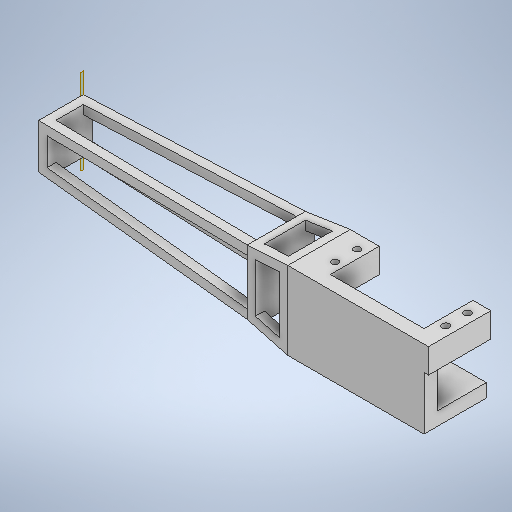
# Autodesk Inventor part: tibiaModel
Saved by Autodesk Inventor 2025.1 (Build 291241020, 241B)
## iProperties
Created: 2021-12-15
Part Number: tibiaModel
Material: 钢
Document SubType Name: Modeling
Designer: omiye
Density: 7.85 g/cm^3
Appearance: Default
Mass: 171.923 g
Surface Area: 96.234 cm^2
Volume: 21.901 cm^3
Sending System: Autodesk Translation Framework v10.10.0.1391
Preprocessor: ST-DEVELOPER v18.1
Title: C:/Users/23714/Desktop/Servo Motor MG996R_ 一字摇臂.step
Autodesk Inventor part; units mm, degrees
ref_plane "YZ Plane" through (0, 0, 0) normal (1, 0, 0) x (0, 1, 0)
ref_plane "XZ Plane" through (0, 0, 0) normal (0, 1, 0) x (-1, 0, 0)
ref_plane "XY Plane" through (0, 0, 0) normal (0, 0, 1) x (1, 0, 0)
ref_plane "Work Plane1" through (-19.25, -0.5, 9.85) normal (0, 0, 1) x (1, 0, 0)
sketch "Sketch1" plane through (-19.25, -0.5, 9.85) normal (0, 0, 1) x (1, 0, 0)
  line L0 (-0.695, -27.8) -> (39.2, -27.8)
  line L1 (39.2, -27.8) -> (39.2, 8.9608)
  line L2 (39.2, 8.9608) -> (-0.695, 8.9608)
  line L3 (-0.695, 8.9608) -> (-0.695, -27.8)
  point P0 (19.25, 0.5)
  constraints: 8 end point, 2 parallel, 1 horizontal, 1 perpendicular
extrude "Extrusion1" add sketch "Sketch1" along normal blind 3
ref_plane "Work Plane2" through (-19.25, -0.5, 12.85) normal (0, 0, 1) x (1, 0, 0)
sketch "Sketch2" plane through (-19.25, -0.5, 12.85) normal (0, 0, 1) x (1, 0, 0)
  line L0 (39.2, -27.8) -> (39.2, 8.9608) projected
  line L1 (39.2, -27.8) -> (-0.695, -27.8)
  line L2 (-0.695, -27.8) -> (-0.695, 8.9608)
  line L3 (-0.695, 8.9608) -> (39.2, 8.9608)
  line L4 (39.2, 8.9608) -> (39.2, -27.8)
  point P0 (19.25, 0.5)
  point P1 (39.2, 8.9608)
  constraints: 8 end point, 2 parallel, 1 horizontal, 1 perpendicular
extrude "Extrusion2" add sketch "Sketch2" along normal blind 5
ref_plane "Work Plane4" through (19.95, -28.3, 9.85) normal (1, 0, 0) x (0, 0, -1)
sketch "Sketch3" plane through (19.95, -28.3, 9.85) normal (1, 0, 0) x (0, 0, -1)
  line L0 (0, 0) -> (0, 36.7608) projected
  line L1 (0, 0) -> (-8, 0) projected
  line L2 (0, 36.7608) -> (-2, 36.7608)
  line L3 (-2, 36.7608) -> (-2, 0)
  line L4 (-2, 0) -> (0, 0)
  line L5 (0, 0) -> (0, 36.7608)
  point P0 (9.85, 28.3)
  dimension "d4" = 2
  constraints: 8 end point, 2 parallel, 1 horizontal, 1 perpendicular, 1 point on line
  measures "d4" distance of L4.end L3.end
extrude "Extrusion3" cut sketch "Sketch3" against normal blind 50
ref_plane "Work Plane3" through (19.95, -28.3, 17.85) normal (1, 0, 0) x (0, 0, -1)
sketch "Sketch4" plane through (19.95, -28.3, 17.85) normal (1, 0, 0) x (0, 0, -1)
  line L0 (6, 0) -> (0, 0) projected
  line L1 (6, 36.7608) -> (0, 36.7608) projected
  line L2 (0, 0) -> (1, 0)
  line L3 (1, 0) -> (1, 36.7608)
  line L4 (1, 36.7608) -> (0, 36.7608)
  line L5 (0, 36.7608) -> (0, 0)
  point P0 (17.85, 28.3)
  point P1 (1, 0)
  dimension "d7" = 1
  constraints: 8 end point, 2 parallel, 1 horizontal, 1 perpendicular, 1 point on line
  measures "d7" distance of L4.end L3.end
extrude "Extrusion4" cut sketch "Sketch4" against normal blind 50
ref_plane "Work Plane5" through (19.95, -28.3, 11.85) normal (1, 0, 0) x (0, 0, -1)
sketch "Sketch5" plane through (19.95, -28.3, 11.85) normal (1, 0, 0) x (0, 0, -1)
  line L0 (-5, 36.7608) -> (-5, 0) projected
  line L1 (0, 0) -> (0, 36.7608) projected
  line L2 (-5, 36.7608) -> (0, 36.7608)
  line L3 (0, 36.7608) -> (0, 0)
  line L4 (0, 0) -> (-5, 0)
  line L5 (-5, 0) -> (-5, 36.7608)
  point P0 (11.85, 28.3)
  constraints: 8 end point, 2 parallel, 1 horizontal, 1 perpendicular
extrude "Extrusion5" add sketch "Sketch5" along normal blind 7
ref_plane "Work Plane6" through (-19.945, -28.3, 11.85) normal (0, 0, -1) x (-1, 0, 0)
sketch "Sketch6" plane through (-19.945, -28.3, 11.85) normal (0, 0, -1) x (-1, 0, 0)
  line L0 (-46.895, 0) -> (-46.895, 36.7608) projected
  line L1 (-46.895, 27.8459) -> (-40.895, 27.8459)
  line L2 (-40.895, 27.8459) -> (-40.895, 11.8459)
  line L3 (-40.895, 11.8459) -> (-46.895, 11.8459)
  line L4 (-46.895, 11.8459) -> (-46.895, 27.8459)
  point P0 (-19.945, 28.3)
  dimension "d12" = 6
  dimension "d13" = 16
  constraints: 8 end point, 2 parallel, 1 horizontal, 1 perpendicular, 1 point on line
  measures "d12" distance of L2.end L3.end
  measures "d13" distance of L1.end L2.end
extrude "Extrusion6" add sketch "Sketch6" along normal blind 22.875
sketch "Sketch7" plane through (20.95, -0.4541, 11.85) normal (0, 1, 0) x (1, 0, 0)
  arc A0 (5.4164, 8.2173) -> (5.4164, 5.6327) centre (3.7611, 6.925) ccw projected
  circle A1 centre (3.7611, 6.925) radius 2.5
  arc A2 (5.4164, 18.0673) -> (5.4164, 15.4827) centre (3.7611, 16.775) ccw projected
  circle A3 centre (3.7611, 16.775) radius 2.5
  point P0 (-20.95, 11.85)
  dimension "d16" = 5
  dimension "d17" = 5
  constraints: 2 centre point, 2 coincident
  measures "d16" diameter of A1
  measures "d17" diameter of A3
extrude "Extrusion7" cut sketch "Sketch7" against normal blind 22.875
ref_plane "Work Plane7" through (26.95, -28.3, 11.85) normal (1, 0, 0) x (0, 0, -1)
sketch "Sketch8" plane through (26.95, -28.3, 11.85) normal (1, 0, 0) x (0, 0, -1)
  line L0 (0, 11.8459) -> (22.875, 11.8459) projected
  line L1 (22.875, 27.8459) -> (22.875, 11.8459) projected
  line L2 (0, 11.8459) -> (22.875, 11.8459)
  line L3 (22.875, 11.8459) -> (22.875, 16.8459)
  line L4 (22.875, 16.8459) -> (0, 16.8459)
  line L5 (0, 16.8459) -> (0, 11.8459)
  point P0 (11.85, 28.3)
  dimension "d20" = 5
  constraints: 8 end point, 2 parallel, 1 horizontal, 1 perpendicular, 1 point on line
  measures "d20" distance of L3.end L2.end
extrude "Extrusion8" cut sketch "Sketch8" against normal blind 6.7
ref_plane "Work Plane8" through (-19.945, -28.3, 11.85) normal (-1, 0, 0) x (0, 0, 1)
sketch "Sketch9" plane through (-19.945, -28.3, 11.85) normal (-1, 0, 0) x (0, 0, 1)
  line L0 (0, 36.7608) -> (0, 0) projected
  line L1 (5, 0) -> (0, 0) projected
  line L2 (0, 36.7608) -> (5, 36.7608)
  line L3 (5, 36.7608) -> (5, 0)
  line L4 (5, 0) -> (0, 0)
  line L5 (0, 0) -> (0, 36.7608)
  point P0 (-11.85, 28.3)
  constraints: 8 end point, 2 parallel, 1 horizontal, 1 perpendicular
extrude "Extrusion9" add sketch "Sketch9" along normal blind 7
ref_plane "Work Plane10" through (26.95, -0.4541, 11.85) normal (0, 0, -1) x (-1, 0, 0)
sketch "Sketch11" plane through (26.95, -0.4541, 11.85) normal (0, 0, -1) x (-1, 0, 0)
  line L0 (53.895, -27.8459) -> (53.895, 8.9148) projected
  line L1 (53.895, 0) -> (47.895, 0)
  line L2 (47.895, 0) -> (47.895, -11)
  line L3 (47.895, -11) -> (53.895, -11)
  line L4 (53.895, -11) -> (53.895, 0)
  point P0 (26.95, 0.4541)
  dimension "d25" = 6
  constraints: 8 end point, 2 parallel, 1 horizontal, 1 perpendicular, 1 point on line
  measures "d25" distance of L3.end L2.end
extrude "Extrusion10" add sketch "Sketch11" along normal blind 22.875
sketch "Sketch12" plane through (-26.945, -0.4541, 11.85) normal (0, 1, 0) x (1, 0, 0)
  arc A0 (0.5786, 15.4827) -> (0.5786, 18.0673) centre (2.2339, 16.775) ccw projected
  circle A1 centre (2.2339, 16.775) radius 2.5
  arc A2 (0.5786, 5.6327) -> (0.5786, 8.2173) centre (2.2339, 6.925) ccw projected
  circle A3 centre (2.2339, 6.925) radius 2.5
  point P0 (26.945, 11.85)
  dimension "d28" = 5
  dimension "d29" = 5
  constraints: 2 centre point, 2 coincident
  measures "d28" diameter of A1
  measures "d29" diameter of A3
extrude "Extrusion11" cut sketch "Sketch12" against normal blind 22.875
ref_plane "Work Plane11" through (-26.945, -28.3, 11.85) normal (-1, 0, 0) x (0, 0, 1)
sketch "Sketch13" plane through (-26.945, -28.3, 11.85) normal (-1, 0, 0) x (0, 0, 1)
  line L0 (0, 16.8459) -> (0, 27.8459) projected
  line L1 (5, 36.7608) -> (0, 36.7608) projected
  line L2 (0, 27.8459) -> (5, 27.8459)
  line L3 (5, 27.8459) -> (5, 36.7608)
  line L4 (5, 36.7608) -> (0, 36.7608)
  line L5 (0, 36.7608) -> (0, 27.8459)
  point P0 (-11.85, 28.3)
  constraints: 8 end point, 2 parallel, 1 horizontal, 1 perpendicular
extrude "Extrusion12" cut sketch "Sketch13" against normal blind 67.325
ref_plane "Work Plane9" through (26.95, -28.3, 11.85) normal (0, -1, 0) x (1, 0, 0)
sketch "Sketch14" plane through (26.95, -28.3, 11.85) normal (0, -1, 0) x (1, 0, 0)
  line L0 (0, 5) -> (0, 0) projected
  line L1 (0, 5) -> (-53.895, 5) projected
  line L2 (0, 0) -> (-53.895, 0)
  line L3 (-53.895, 0) -> (-53.895, 5)
  line L4 (-53.895, 5) -> (0, 5)
  line L5 (0, 5) -> (0, 0)
  point P0 (-26.95, -11.85)
  constraints: 8 end point, 2 parallel, 1 horizontal, 1 perpendicular
extrude "Extrusion13" add sketch "Sketch14" along normal blind 5
ref_plane "Work Plane12" through (26.95, -11.4541, 11.85) normal (0, 0, -1) x (-1, 0, 0)
sketch "Sketch15" plane through (26.95, -11.4541, 11.85) normal (0, 0, -1) x (-1, 0, 0)
  line L0 (53.895, -21.8459) -> (0, -21.8459) projected
  line L1 (53.895, 11) -> (53.895, -21.8459) projected
  line L2 (0, -21.8459) -> (53.895, -21.8459)
  line L3 (53.895, -21.8459) -> (53.895, -17.8459)
  line L4 (53.895, -17.8459) -> (0, -17.8459)
  line L5 (0, -17.8459) -> (0, -21.8459)
  point P0 (26.95, 11.4541)
  dimension "d36" = 4
  constraints: 8 end point, 2 parallel, 1 horizontal, 1 perpendicular, 1 point on line
  measures "d36" distance of L3.end L2.end
extrude "Extrusion14" add sketch "Sketch15" along normal blind 22.4625
ref_plane "Work Plane13" through (-26.945, -29.3, 11.85) normal (0, 1, 0) x (1, 0, 0)
sketch "Sketch16" plane through (-26.945, -29.3, 11.85) normal (0, 1, 0) x (1, 0, 0)
  line L0 (53.895, 0) -> (53.895, 22.4625) projected
  line L1 (0, 0) -> (0, 22.4625) projected
  line L2 (53.895, 0) -> (0, 0)
  line L3 (0, 0) -> (0, 1)
  line L4 (0, 1) -> (53.895, 1)
  line L5 (53.895, 1) -> (53.895, 0)
  point P0 (26.945, 11.85)
  point P1 (53.895, 1)
  dimension "d39" = 1
  constraints: 8 end point, 2 parallel, 1 horizontal, 1 perpendicular, 1 point on line
  measures "d39" distance of L2.end L3.end
extrude "Extrusion15" add sketch "Sketch16" along normal blind 30
ref_plane "Work Plane14" through (26.95, -28.3, 11.85) normal (1, 0, 0) x (0, 0, -1)
sketch "Sketch17" plane through (26.95, -28.3, 11.85) normal (1, 0, 0) x (0, 0, -1)
  line L0 (0, 29) -> (1, 29) projected
  line L1 (5.8126, 27.8459) -> (1, 27.8459) projected
  line L2 (0, 29) -> (1, 29)
  line L3 (1, 29) -> (1, 27.8459)
  line L4 (1, 27.8459) -> (0, 27.8459)
  line L5 (0, 27.8459) -> (0, 29)
  point P0 (11.85, 28.3)
  constraints: 8 end point, 2 parallel, 1 horizontal, 1 perpendicular
extrude "Extrusion16" cut sketch "Sketch17" against normal blind 100
sketch "Sketch19" plane through (26.95, -33.3, 11.85) normal (0, -1, 0) x (1, 0, 0)
  circle A0 centre (-16.85, -11.85) radius 5
  circle A1 centre (-16.85, -11.85) radius 1.5
  point P0 (-26.95, -11.85)
  dimension "d47" = 10
  dimension "d50" = 3
  constraints: 2 centre point, 1 coincident
  measures "d47" diameter of A0
  measures "d50" diameter of A1
extrude "Extrusion20" cut sketch "Sketch19" against normal blind 10 contours A1
sketch "Sketch20" plane through (26.95, -33.3, 11.85) normal (0, -1, 0) x (1, 0, 0)
  line L0 (-53.895, -22.4625) -> (0, -22.4625) projected
  line L1 (-53.895, 5) -> (-53.895, -22.4625) projected
  line L2 (0, -22.4625) -> (-53.895, -22.4625)
  line L3 (-53.895, -22.4625) -> (-53.895, 5)
  line L4 (-53.895, 5) -> (0, 5)
  line L5 (0, 5) -> (0, -22.4625)
  point P0 (-26.95, -11.85)
  constraints: 8 end point, 2 parallel, 1 horizontal, 1 perpendicular
extrude "Extrusion21" add sketch "Sketch20" along normal blind 2
sketch "Sketch21" plane through (-26.945, -29.3, -10.6125) normal (0, 1, 0) x (1, 0, 0)
  circle A0 centre (37.045, -10.6125) radius 1.5 projected
  circle A1 centre (37.045, -10.6125) radius 1.5
  point P0 (26.945, -10.6125)
  constraints: 1 centre point, 1 coincident
extrude "Extrusion22" cut sketch "Sketch21" against normal blind 10
sketch "Sketch22" plane through (-26.945, -29.3, -10.6125) normal (0, 1, 0) x (1, 0, 0)
  circle A0 centre (37.045, -10.6125) radius 1.5 projected
  circle A1 centre (37.045, -10.6125) radius 2.5
  point P0 (26.945, -10.6125)
  dimension "d59" = 5
  constraints: 1 centre point, 1 coincident
  measures "d59" diameter of A1
extrude "Extrusion23" cut sketch "Sketch22" against normal blind 2
sketch "Sketch23" plane through (-19.945, -28.3, -11.025) normal (0, 0, -1) x (-1, 0, 0)
  line L0 (-46.895, 27.8459) -> (-46.895, 16.8459) projected
  line L1 (-46.895, 27.8459) -> (-48.895, 27.8459)
  line L2 (-48.895, 27.8459) -> (-48.895, 16.8459)
  line L3 (-48.895, 16.8459) -> (-46.895, 16.8459)
  line L4 (-46.895, 16.8459) -> (-46.895, 27.8459)
  line L5 (7, 16.8459) -> (7, 27.8459) projected
  line L6 (7, 27.8459) -> (9, 27.8459)
  line L7 (9, 27.8459) -> (9, 16.8459)
  line L8 (9, 16.8459) -> (7, 16.8459)
  line L9 (7, 16.8459) -> (7, 27.8459)
  point P0 (-19.945, 28.3)
  dimension "d62" = 2
  dimension "d63" = 2
  constraints: 16 end point, 4 parallel, 2 horizontal, 2 perpendicular, 1 point on line
  measures "d62" distance of L3.end L2.end
  measures "d63" distance of L7.end L8.end
extrude "Extrusion24" add sketch "Sketch23" against normal up to surface (27.875 mm away)
sketch "Sketch24" plane through (-20.945, -0.4541, 10.85) normal (0, 1, 0) x (1, 0, 0)
  arc A0 (47.895, 7.0374) -> (47.895, 4.8126) centre (45.6561, 5.925) ccw projected
  circle A1 centre (45.6561, 5.925) radius 1.6
  arc A2 (47.895, 16.8874) -> (47.895, 14.6626) centre (45.6561, 15.775) ccw projected
  circle A3 centre (45.6561, 15.775) radius 1.6
  circle A4 centre (45.6561, 5.925) radius 2.5
  circle A5 centre (45.6561, 15.775) radius 2.5
  point P0 (20.945, 10.85)
  point P1 (47.895, 4.8126)
  dimension "d66" = 3.2
  dimension "d67" = 3.2
  constraints: 4 centre point, 4 coincident
  measures "d66" diameter of A1
  measures "d67" diameter of A3
extrude "Extrusion25" add sketch "Sketch24" against normal up to surface (11 mm away)
sketch "Sketch25" plane through (-20.945, -0.4541, 10.85) normal (0, 1, 0) x (1, 0, 0)
  arc A0 (-6, 4.8025) -> (-6, 7.0475) centre (-3.7661, 5.925) ccw projected
  circle A1 centre (-3.7661, 5.925) radius 1.6
  arc A2 (-6, 14.6525) -> (-6, 16.8975) centre (-3.7661, 15.775) ccw projected
  circle A3 centre (-3.7661, 15.775) radius 1.6
  circle A4 centre (-3.7661, 15.775) radius 2.5
  circle A5 centre (-3.7661, 5.925) radius 2.5
  point P0 (20.945, 10.85)
  point P1 (-6, 7.0475)
  dimension "d70" = 3.2
  dimension "d71" = 3.2
  dimension "d72" = 5
  dimension "d73" = 5
  constraints: 4 centre point, 4 coincident
  measures "d70" diameter of A1
  measures "d71" diameter of A3
  measures "d72" diameter of A4
  measures "d73" diameter of A5
extrude "Extrusion26" add sketch "Sketch25" against normal up to surface (11 mm away)
sketch "Sketch26" plane through (-20.945, -0.4541, 10.85) normal (0, 1, 0) x (1, 0, 0)
  circle A0 centre (-3.7661, 15.775) radius 1.6 projected
  circle A1 centre (-3.7661, 15.775) radius 1.6
  circle A2 centre (-3.7661, 15.775) radius 1.5
  circle A3 centre (-3.7661, 5.925) radius 1.6 projected
  circle A4 centre (-3.7661, 5.925) radius 1.5
  point P0 (20.945, 10.85)
  dimension "d76" = 3
  dimension "d77" = 3
  constraints: 3 centre point, 3 coincident
  measures "d76" diameter of A2
  measures "d77" diameter of A4
extrude "Extrusion27" add sketch "Sketch26" against normal up to surface (11 mm away)
sketch "Sketch27" plane through (-26.945, -28.3, 11.85) normal (-1, 0, 0) x (0, 0, 1)
  line L0 (5, 16.8459) -> (5, -7) projected
  line L1 (-1, -1) -> (-22.4625, -1) projected
  line L2 (5, 16.8459) -> (-1, 16.8459)
  line L3 (-1, 16.8459) -> (-1, -1)
  line L4 (-1, -1) -> (5, -1)
  line L5 (5, -1) -> (5, 16.8459)
  line L6 (-22.4625, -7) -> (5, -7) projected
  line L7 (5, -1) -> (-22.4625, -1)
  line L8 (-22.4625, -1) -> (-22.4625, -7)
  line L9 (-22.4625, -7) -> (5, -7)
  line L10 (5, -7) -> (5, -1)
  point P0 (-11.85, 28.3)
  constraints: 16 end point, 4 parallel, 2 horizontal, 2 perpendicular
extrude "Extrusion28" add sketch "Sketch27" along normal up to surface (2 mm away)
sketch "Sketch28" plane through (-28.945, -11.4541, -11.025) normal (-1, 0, 0) x (0, 0, 1)
  line L0 (21.875, 11) -> (0, 11) projected
  line L1 (0.4125, -23.8459) -> (27.875, -23.8459) projected
  line L2 (0, 11) -> (27.875, 11)
  line L3 (27.875, 11) -> (27.875, -23.8459)
  line L4 (27.875, -23.8459) -> (0, -23.8459)
  line L5 (0, -23.8459) -> (0, 11)
  point P0 (11.025, 11.4541)
  constraints: 8 end point, 2 parallel, 1 horizontal, 1 perpendicular
extrude "Extrusion29" add sketch "Sketch28" along normal blind 5
sketch "Sketch29" plane through (26.95, -11.4541, -10.6125) normal (0, 0, -1) x (-1, 0, 0)
  line L0 (0, -17.8459) -> (0, -23.8459) projected
  line L1 (55.895, -23.8459) -> (60.895, -23.8459) projected
  line L2 (0, -17.8459) -> (55.895, -17.8459)
  line L3 (55.895, -17.8459) -> (55.895, -23.8459)
  line L4 (55.895, -23.8459) -> (0, -23.8459)
  line L5 (0, -23.8459) -> (0, -17.8459)
  point P0 (26.95, 11.4541)
  constraints: 8 end point, 2 parallel, 1 horizontal, 1 perpendicular
extrude "Extrusion30" add sketch "Sketch29" along normal up to surface (0.4125 mm away)
sketch "Sketch30" plane through (10.1, -31.3, 0) normal (0, 1, 0) x (1, 0, 0)
  circle A0 centre (0, 0) radius 1.5 projected
  circle A1 centre (0, 0) radius 2.5
  point P0 (-10.1, 0)
  constraints: 1 centre point, 1 coincident
extrude "Extrusion31" cut sketch "Sketch30" against normal blind 1
sketch "Sketch32" plane through (-20.945, -0.4541, 10.85) normal (0, 1, 0) x (1, 0, 0)
  line L0 (47.895, 21.875) -> (-13, 21.875) projected
  line L1 (-13, 21.875) -> (7, 21.875) construction
  line L2 (49.895, -6) -> (-13, -6) projected
  line L3 (-92.0124, 9.713) -> (-92.0124, 6.162)
  line L4 (-13, 21.875) -> (-13, -6) projected
  line L5 (-13, 21.875) -> (-33, 21.875)
  line L6 (-13, -6) -> (-13, 21.875)
  line L7 (-33, 21.875) -> (-33, -6)
  line L8 (-13, -6) -> (-33, -4.2502)
  line L9 (-13, -6) -> (7.0764, -6) construction
  line L10 (-13, -6) -> (-13, 21.875)
  line L11 (-13, -6) -> (-13, 21.875)
  line L12 (-13, 21.875) -> (-18, 21.875)
  line L13 (-18, 21.875) -> (-18, -6)
  line L14 (-18, -6) -> (-13, -6)
  line L15 (-13, 21.875) -> (-33, 21.875)
  line L16 (-33, 21.875) -> (-33, 16.875)
  line L17 (-33, 16.875) -> (-13, 16.875)
  line L18 (-13, 16.875) -> (-13, 21.875)
  line L19 (-33, 21.875) -> (-33, -4.2502)
  line L20 (-33, -4.2502) -> (-28, -4.2502)
  line L21 (-28, -4.2502) -> (-28, 21.875)
  line L22 (-28, 21.875) -> (-33, 21.875)
  line L23 (-13, -6) -> (-33, -4.2502)
  line L24 (-33, -4.2502) -> (-32.5642, 0.7307)
  line L25 (-32.5642, 0.7307) -> (-12.5642, -1.019)
  line L26 (-12.5642, -1.019) -> (-13, -6)
  line L27 (-13, 16.875) -> (-33, 16.875)
  line L28 (-32.5642, 0.7307) -> (-33, 0.7307)
  point P0 (20.945, 10.85)
  point P1 (-18, 16.875)
  point P2 (-18, -0.5435)
  point P3 (-28, 0.3314)
  point P4 (-28, 16.875)
  dimension "d101" = 175
  dimension "d102" = 5
  dimension "d103" = 5
  dimension "d104" = 5
  dimension "d105" = 5
  constraints: 52 end point, 9 parallel, 5 collinear, 5 perpendicular, 3 horizontal, 3 vertical, 2 point on line, 1 equal length
  measures "d101" angle of L9 L8
  measures "d102" distance of L12.end L0.end
  measures "d103" distance of L16.end L5.end
  measures "d104" distance of L20.end L8.end
  measures "d105" distance of L8.end L24.end
extrude "Extrusion32" add sketch "Sketch32" against normal up to surface (34.8459 mm away) contours L4 L17 L13 L5 | L4 L25 L13 L17 | L13 L17 L21 L5 | L4 L8 L13 L25 | L21 L17 L7 L5 | L13 L8 L20 L21 L25 | L21 L25 L28 L7 L17 | L21 L20 L24 L25 | L7 L28 L24
sketch "Sketch33" plane through (-20.945, -0.4541, 10.85) normal (0, 1, 0) x (1, 0, 0)
  line L0 (-33, -4.2502) -> (-13, -6) projected
  line L1 (-33, -4.2502) -> (-101.9365, 7.9051)
  line L2 (-33, -4.2502) -> (37, -4.2502) construction
  line L3 (-33, 21.875) -> (0, 21.875) projected
  line L4 (-33, 21.875) -> (-101.9365, 21.875)
  line L5 (-33, 21.875) -> (35.9365, 21.875) construction
  line L6 (-101.9365, 21.875) -> (-101.9365, 7.9051)
  line L7 (-33, -4.2502) -> (-33, 21.875)
  line L8 (-33, 21.875) -> (-38, 21.875)
  line L9 (-38, 21.875) -> (-38, -4.2502)
  line L10 (-38, -4.2502) -> (-33, -4.2502)
  line L11 (-33, -4.2502) -> (-101.9365, 7.9051)
  line L12 (-101.9365, 7.9051) -> (-101.0683, 12.8292)
  line L13 (-101.0683, 12.8292) -> (-32.1318, 0.6738)
  line L14 (-32.1318, 0.6738) -> (-33, -4.2502)
  line L15 (-101.9365, 21.875) -> (-101.9365, 7.9051)
  line L16 (-101.9365, 7.9051) -> (-96.9365, 7.9051)
  line L17 (-96.9365, 7.9051) -> (-96.9365, 21.875)
  line L18 (-96.9365, 21.875) -> (-101.9365, 21.875)
  line L19 (-101.9365, 21.875) -> (-33, 21.875)
  line L20 (-33, 21.875) -> (-33, 16.875)
  line L21 (-33, 16.875) -> (-101.9365, 16.875)
  line L22 (-101.9365, 16.875) -> (-101.9365, 21.875)
  point P0 (20.945, 10.85)
  point P1 (-33, 0.8269)
  point P2 (-96.9365, 12.1006)
  point P3 (-96.9365, 16.875)
  dimension "d108" = 70
  dimension "d109" = 170
  dimension "d110" = 180
  dimension "d111" = 5
  dimension "d112" = 5
  dimension "d113" = 5
  dimension "d114" = 5
  constraints: 42 end point, 12 equal length, 5 perpendicular, 2 horizontal
  measures "d108" distance of L0.start L1.end
  measures "d109" angle of L2 L1
  measures "d110" angle of L4 L5
  measures "d111" distance of L8.end L3.start
  measures "d112" distance of L1.end L12.end
  measures "d113" distance of L16.end L1.end
  measures "d114" distance of L3.start L20.end
extrude "Extrusion33" add sketch "Sketch33" against normal up to surface (34.8459 mm away) contours L1 L9 L13 L7 | L1 L16 L17 L13 L9 | L6 L21 L17 L13 L12 | L12 L13 L17 L16 | L21 L9 L4 L7 | L6 L4 L17 L21 | L21 L17 L4 L9
sketch "Sketch34" plane through (-20.945, -0.4541, 10.85) normal (0, 1, 0) x (1, 0, 0)
  line L0 (-101.9365, 7.9051) -> (-101.9365, 21.875) projected
  line L1 (-101.9365, 7.9051) -> (-117.2574, 20.7609)
  line L2 (-101.9365, 7.9051) -> (-81.9365, 7.9051) construction
  line L3 (-117.2574, 20.7609) -> (-117.2574, 22.7609)
  line L4 (-117.2574, 22.7609) -> (-101.9365, 21.875)
  line L5 (-101.9365, 7.9051) -> (-118.8375, 22.0867)
  line L6 (-118.8375, 22.0867) -> (-116.5877, 24.7679)
  line L7 (-116.5877, 24.7679) -> (-99.6868, 10.5863)
  line L8 (-99.6868, 10.5863) -> (-101.9365, 7.9051)
  line L9 (-101.9365, 21.875) -> (0, 21.875) projected
  line L10 (-117.2574, 22.7609) -> (-101.6974, 21.875)
  line L11 (-101.6974, 21.875) -> (-101.8963, 18.3807)
  line L12 (-101.8963, 18.3807) -> (-117.4564, 19.2666)
  line L13 (-117.4564, 19.2666) -> (-117.2574, 22.7609)
  point P0 (20.945, 10.85)
  point P1 (-101.9365, 12.4741)
  point P2 (-109.4911, 18.8131)
  point P3 (-101.9365, 18.3829)
  point P4 (-117.3661, 20.8521)
  point P5 (-117.2574, 20.7609)
  dimension "d117" = 20
  dimension "d118" = 140
  dimension "d119" = 2
  dimension "d120" = 3.5
  dimension "d121" = 3.5
  constraints: 24 end point, 5 parallel, 2 perpendicular, 2 point on line, 1 equal length, 1 horizontal
  measures "d117" distance of L0.start L1.end
  measures "d118" angle of L2 L1
  measures "d119" distance of L1.end L3.end
  measures "d120" distance of L5.end L6.end
  measures "d121" distance of L10.end L11.end
extrude "Extrusion34" add sketch "Sketch34" against normal up to surface (34.8459 mm away) contours L1 L12 L7 L0 | L1 L3 L4 L7 L12 | L12 L7 L4 L0 | L5 L13 L3
sketch "Sketch35" plane through (-20.945, -0.4541, 10.85) normal (0, 1, 0) x (1, 0, 0)
  line L0 (-117.2574, 22.7609) -> (-101.9365, 21.875) projected
  line L1 (-101.9365, 21.875) -> (-117.3079, 21.875)
  line L2 (-117.3661, 20.8521) -> (-117.2574, 22.7609) projected
  line L3 (-101.9365, 21.875) -> (-86.5652, 21.875) construction
  line L4 (-101.9365, 21.875) -> (-117.2574, 22.7609)
  line L5 (-117.3079, 21.875) -> (-117.2574, 22.7609)
  point P0 (20.945, 10.85)
  dimension "d124" = 180
  constraints: 8 end point, 3 collinear, 1 horizontal, 1 point on line
  measures "d124" angle of L1 L3
extrude "Extrusion35" cut sketch "Sketch35" against normal blind 46.5125
sketch "Sketch36" plane through (-20.945, -0.4541, 10.85) normal (0, 1, 0) x (1, 0, 0)
  line L0 (-117.3079, 21.875) -> (-101.9365, 21.875) projected
  line L1 (-117.3079, 21.875) -> (-117.3079, 20.8032)
  line L2 (-101.9365, 7.9051) -> (-117.3661, 20.8521) projected
  line L3 (-117.3079, 21.875) -> (-117.3661, 20.8521) projected
  line L4 (-117.3079, 20.8032) -> (-117.3661, 20.8521)
  point P0 (20.945, 10.85)
  point P1 (-33, 21.875)
  constraints: 4 end point, 1 point on line, 1 vertical
extrude "Extrusion36" cut sketch "Sketch36" against normal blind 44.925
sketch "Sketch38" plane through (26.95, -0.4541, -11.025) normal (0, 0, -1) x (-1, 0, 0)
  line L0 (47.895, -11) -> (55.895, -11) projected
  line L1 (0, -28.8459) -> (55.895, -28.8459) projected
  line L2 (55.895, -11) -> (55.895, -28.8459)
  line L3 (55.895, -28.8459) -> (58.895, -28.8459)
  line L4 (58.895, -28.8459) -> (58.895, -11)
  line L5 (58.895, -11) -> (55.895, -11)
  point P0 (26.95, 0.4541)
  dimension "d132" = 3
  constraints: 8 end point, 2 parallel, 2 perpendicular
  measures "d132" distance of L3.end L1.end
extrude "Extrusion38" cut sketch "Sketch38" against normal up to surface (21.875 mm away)
sketch "Sketch39" plane through (26.95, -35.3, 11.85) normal (0, -1, 0) x (1, 0, 0)
  line L0 (-80.895, 3.2502) -> (-60.895, 5) projected
  line L1 (-165.2029, -22.875) -> (-47.895, -22.875) projected
  line L2 (-60.895, 5) -> (-60.895, -22.875)
  line L3 (-60.895, -22.875) -> (-165.2029, -22.875)
  line L4 (-165.2029, -22.875) -> (-165.2029, 5)
  line L5 (-165.2029, 5) -> (-60.895, 5)
  line L6 (-165.2029, -22.875) -> (-165.2029, 5)
  line L7 (-165.2029, 5) -> (-180.2029, 5)
  line L8 (-180.2029, 5) -> (-180.2029, -22.875)
  line L9 (-180.2029, -22.875) -> (-165.2029, -22.875)
  point P0 (-26.95, -11.85)
  dimension "d135" = 15
  constraints: 16 end point, 5 equal length, 2 perpendicular, 1 point on line, 1 vertical
  measures "d135" distance of L7.end L4.end
ref_plane "Work Plane15" through (-153.2529, -0.4541, -11.025) normal (-1, 0, 0) x (0, 0, 1)
sketch "Sketch40" plane through (-153.2529, -0.4541, -11.025) normal (-1, 0, 0) x (0, 0, 1)
  line L0 (0, 0) -> (0, -34.8459) projected
  line L1 (0, -11) -> (0, 0) projected
  line L2 (0, -34.8459) -> (0, 0)
  line L3 (0, 0) -> (0, -17.423)
  line L4 (0, -17.423) -> (0, -27.423)
  line L5 (0, -17.423) -> (10, -17.423) construction
  line L6 (0, -27.423) -> (0, -7.423)
  line L7 (0, -7.423) -> (20, -7.423)
  line L8 (20, -7.423) -> (20, -27.423)
  line L9 (20, -27.423) -> (0, -27.423)
  circle A0 centre (10, -17.423) radius 10
  point P0 (11.025, 0.4541)
  dimension "d137" = 10
  dimension "d138" = 90
  dimension "d139" = 20
  dimension "d140" = 20
  dimension "d141" = 20
  constraints: 16 end point, 2 parallel, 2 perpendicular, 1 centre point, 1 coincident, 1 collinear, 1 horizontal, 1 midpoint, 1 point on line, 1 vertical
  measures "d137" distance of L3.end L4.end
  measures "d138" angle of L4 L5
  measures "d139" distance of L4.end L6.end
  measures "d140" distance of L6.end L7.end
  measures "d141" diameter of A0
sketch "Sketch42" plane through (-53.945, -0.4541, -6.025) normal (-1, 0, 0) x (0, 0, 1)
  line L0 (-5, -34.8459) -> (-5, -31.8459)
  line L1 (-5, -31.8459) -> (-5, 0)
  line L2 (-5, 0) -> (-5, -3)
  line L3 (-5, -3) -> (-5, -31.8459)
  line L4 (-5, -31.8459) -> (-5, -3)
  line L5 (-5, -3) -> (21, -3)
  line L6 (21, -3) -> (21, -31.8459)
  line L7 (21, -31.8459) -> (-5, -31.8459)
  line L8 (12.55, -11) -> (12.55, 0) projected
  point P0 (6.025, 0.4541)
  dimension "d146" = 3
  dimension "d147" = 3
  dimension "d148" = 26
  constraints: 16 end point, 3 parallel, 1 collinear, 1 perpendicular, 1 point on line, 1 vertical
  measures "d146" distance of L0.start L0.end
  measures "d147" distance of L1.end L2.end
  measures "d148" distance of L2.end L5.end
extrude "Extrusion39" cut sketch "Sketch39" against normal blind 45.5625 contours L4 L5 L2 L1
loft "Loft1" add profiles "Sketch42" section 1 edges at (-33.945, -0.4541, 2.9125) (-33.945, -17.877, -11.025) (-33.945, -35.3, 2.9125) (-33.945, -17.877, 16.85)
loft "Loft2" add profiles "Sketch40" section 1 edges at (-53.945, -3.4541, 1.975) (-53.945, -17.877, -11.025) (-53.945, -32.3, 1.975) (-53.945, -17.877, 14.975)
sketch "Sketch43" plane through (26.95, -0.4541, -11.025) normal (0, 0, -1) x (-1, 0, 0)
  line L0 (60.895, 0) -> (80.895, -3) projected
  line L1 (60.895, -34.8459) -> (80.895, -31.8459) projected
  line L2 (80.895, -3) -> (80.895, -31.8459)
  line L3 (80.895, -31.8459) -> (76.895, -31.8459)
  line L4 (80.895, -31.8459) -> (80.3016, -27.8902)
  line L5 (60.895, -34.8459) -> (60.895, 0) projected
  line L6 (60.895, -34.8459) -> (60.895, 0)
  line L7 (60.895, 0) -> (64.895, 0)
  line L8 (60.895, -34.8459) -> (64.895, -34.8459)
  line L9 (64.895, -34.8459) -> (64.895, -0.6)
  line L10 (64.895, -34.2459) -> (60.895, -34.2459)
  line L11 (64.895, -0.6) -> (60.895, -0.6)
  line L12 (60.895, -34.2459) -> (60.895, -0.6)
  line L13 (76.895, -31.8459) -> (76.895, -3)
  line L14 (80.895, -3) -> (76.895, -3)
  line L15 (64.895, -34.2459) -> (80.895, -31.8459)
  line L16 (80.895, -31.8459) -> (80.3016, -27.8902)
  line L17 (80.3016, -27.8902) -> (64.3016, -30.2902)
  line L18 (64.3016, -30.2902) -> (64.895, -34.2459)
  line L19 (80.895, -3) -> (64.895, -0.6)
  line L20 (64.895, -0.6) -> (64.3016, -4.5557)
  line L21 (64.3016, -4.5557) -> (80.3016, -6.9557)
  line L22 (80.3016, -6.9557) -> (80.895, -3)
  line L23 (64.895, -30.2012) -> (76.895, -28.4012)
  line L24 (76.895, -28.4012) -> (76.895, -6.4447)
  line L25 (76.895, -6.4447) -> (64.895, -4.6447)
  line L26 (64.895, -4.6447) -> (64.895, -30.2012)
  point P0 (26.95, 0.4541)
  dimension "d159" = 4
  dimension "d160" = 4
  dimension "d161" = 4
  dimension "d162" = 4
  dimension "d163" = 4
  dimension "d164" = 4
  constraints: 48 end point, 13 point on line, 7 perpendicular, 5 collinear, 5 parallel, 3 horizontal, 1 vertical
  measures "d159" distance of L1.end L3.end
  measures "d160" distance of L1.end L4.end
  measures "d161" distance of L0.start L7.end
  measures "d162" distance of L1.start L8.end
  measures "d163" distance of L16.end L1.end
  measures "d164" distance of L20.end L9.end
extrude "Extrusion40" cut sketch "Sketch43" against normal blind 45.5625 contours L21 L13 L17 L9
sketch "Sketch44" plane through (26.95, -35.3, 11.85) normal (0, -1, 0) x (1, 0, 0)
  line L0 (-60.895, 5) -> (-80.895, 3.125) projected
  line L1 (-60.895, -22.875) -> (-60.895, 5) projected
  line L2 (-60.895, 5) -> (-60.895, -22.875)
  line L3 (-60.895, -22.875) -> (-64.895, -22.875)
  line L4 (-64.895, -22.875) -> (-64.895, 5)
  line L5 (-64.895, 5) -> (-60.895, 5)
  line L6 (-80.895, 3.125) -> (-80.895, -22.875) projected
  line L7 (-80.895, -22.875) -> (-80.895, 3.125)
  line L8 (-80.895, 3.125) -> (-76.895, 3.125)
  line L9 (-76.895, 3.125) -> (-76.895, -22.875)
  line L10 (-76.895, -22.875) -> (-80.895, -22.875)
  line L11 (-60.895, 5) -> (-80.895, 3.125)
  line L12 (-80.895, 3.125) -> (-80.5216, -0.8575)
  line L13 (-80.5216, -0.8575) -> (-60.5216, 1.0175)
  line L14 (-60.5216, 1.0175) -> (-60.895, 5)
  line L15 (-80.895, -22.875) -> (-60.895, -22.875)
  line L16 (-60.895, -22.875) -> (-60.895, -18.875)
  line L17 (-60.895, -18.875) -> (-80.895, -18.875)
  line L18 (-80.895, -18.875) -> (-80.895, -22.875)
  line L19 (-64.895, 0.6075) -> (-76.895, -0.5175)
  line L20 (-76.895, -0.5175) -> (-76.895, -18.875)
  line L21 (-76.895, -18.875) -> (-64.895, -18.875)
  line L22 (-64.895, -18.875) -> (-64.895, 0.6075)
  point P0 (-26.95, -11.85)
  dimension "d167" = 4
  dimension "d168" = 4
  dimension "d169" = 4
  dimension "d170" = 4
  constraints: 40 end point, 8 parallel, 8 point on line, 4 collinear, 4 perpendicular
  measures "d167" distance of L1.start L3.end
  measures "d168" distance of L0.end L8.end
  measures "d169" distance of L12.end L0.end
  measures "d170" distance of L16.end L1.start
extrude "Extrusion41" cut sketch "Sketch44" against normal blind 45.5625 contours L4 L17 L9 L13
sketch "Sketch45" plane through (26.95, -0.4541, -11.025) normal (0, 0, -1) x (-1, 0, 0)
  line L0 (80.895, -31.8459) -> (180.2029, -27.423) projected
  line L1 (180.2029, -27.423) -> (80.895, -31.8459)
  line L2 (80.895, -31.8459) -> (80.717, -27.8499)
  line L3 (80.717, -27.8499) -> (180.0249, -23.4269)
  line L4 (180.0249, -23.4269) -> (180.2029, -27.423)
  line L5 (180.2029, -27.423) -> (180.2029, -7.423) projected
  line L6 (80.895, -3) -> (180.2029, -7.423) projected
  line L7 (180.2029, -7.423) -> (80.895, -3)
  line L8 (80.895, -3) -> (80.717, -6.996)
  line L9 (80.717, -6.996) -> (180.0249, -11.419)
  line L10 (180.0249, -11.419) -> (180.2029, -7.423)
  line L11 (180.2029, -27.423) -> (180.2029, -7.423)
  line L12 (180.2029, -7.423) -> (176.2029, -7.423)
  line L13 (176.2029, -7.423) -> (176.2029, -27.423)
  line L14 (176.2029, -27.423) -> (180.2029, -27.423)
  line L15 (80.895, -31.8459) -> (80.895, -3) projected
  line L16 (80.717, -27.8499) -> (80.717, -6.996)
  point P0 (26.95, 0.4541)
  point P1 (80.895, -7.004)
  point P2 (80.895, -27.842)
  point P3 (176.2029, -23.5972)
  point P4 (176.2029, -11.2488)
  dimension "d173" = 4
  dimension "d174" = 4
  dimension "d175" = 4
  constraints: 26 end point, 8 equal length, 3 perpendicular, 1 vertical
  measures "d173" distance of L0.start L2.end
  measures "d174" distance of L8.end L6.start
  measures "d175" distance of L12.end L5.end
extrude "Extrusion42" cut sketch "Sketch45" against normal blind 45.5625 contours L15 L9 L13 L3
sketch "Sketch46" plane through (26.95, -35.3, 11.85) normal (0, -1, 0) x (1, 0, 0)
  line L0 (-180.2029, -2.875) -> (-180.2029, -22.875) projected
  line L1 (-80.895, 3.125) -> (-180.2029, -2.875) projected
  line L2 (-180.2029, -2.875) -> (-80.895, 3.125)
  line L3 (-80.895, 3.125) -> (-80.6538, -0.8677)
  line L4 (-80.6538, -0.8677) -> (-179.9616, -6.8677)
  line L5 (-179.9616, -6.8677) -> (-180.2029, -2.875)
  line L6 (-80.895, -22.875) -> (-180.2029, -22.875) projected
  line L7 (-180.2029, -22.875) -> (-80.895, -22.875)
  line L8 (-80.895, -22.875) -> (-80.895, -18.875)
  line L9 (-80.895, -18.875) -> (-180.2029, -18.875)
  line L10 (-180.2029, -18.875) -> (-180.2029, -22.875)
  line L11 (-180.2029, -2.875) -> (-180.2029, -22.875)
  line L12 (-180.2029, -22.875) -> (-176.2029, -22.875)
  line L13 (-176.2029, -22.875) -> (-176.2029, -2.875)
  line L14 (-176.2029, -2.875) -> (-180.2029, -2.875)
  line L15 (-80.895, -18.875) -> (-80.895, -0.8823)
  line L16 (-80.895, -22.875) -> (-80.895, 3.125) projected
  line L17 (-80.895, -0.8823) -> (-176.2029, -6.6406)
  point P0 (-26.95, -11.85)
  point P1 (-176.2029, -18.875)
  dimension "d178" = 4
  dimension "d179" = 4
  dimension "d180" = 4
  constraints: 28 end point, 6 parallel, 4 point on line, 3 collinear, 3 perpendicular
  measures "d178" distance of L1.start L3.end
  measures "d179" distance of L8.end L6.start
  measures "d180" distance of L12.end L0.end
extrude "Extrusion43" cut sketch "Sketch46" against normal blind 45.5625 contours L13 L4 L15 L9
body "Solid1"
body "Solid13"
